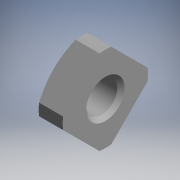
# Autodesk Inventor part: DIN 557 - M4
Saved by Autodesk Inventor 2017.3 (Build 213256000, 256)
## iProperties
Part Number: DIN 557 - M4
Material: Generic
Catalog Web Link: www.cadenas.de
Description: DIN-557-Square nuts
Vendor: FESTO
Document SubType Name: Modeling
Designer: partserver
Manufacturer: FESTO
Mass: 0.122402 g
Surface Area: 1.83702 cm^2
Volume: 0.122402 cm^3
Density: 1 g/cm^3
Appearance: PSOLRGB-192-192-192
Category: PARTsolutions
Company: FESTO
Title: DIN 557 - M4
Author: Cadenas PARTsolutions
Comments: Square nuts
PSOL_IDENT_0: {$CADENAS_DATA\23d-libs\festo\zyl_zubeh\din_557\din_557.prj},178 {VTYP=3D},{NB=DIN 557 - M4},{LINA=D
PSOL_IDENT_1: IN 557 - M4},{NN=DIN-557},{DATE=28.05.2015 11:13:37},{GEOMDATE=10.08.2011 05:48:00},{VERSION=v070619
PSOL_IDENT_2: 081727},{LINEID=10},{WBVAR=},{WBNUMERIC=}  {NB=DIN 557 - M4},{LINA=DIN 557 - M4},{KT=X},{IDNR=},{NEN
PSOL_IDENT_3: N=M4},{D=4.000},{D1=4.134},{P=0.700},{M=3.200},{S=7.000},{SW=},{DW=5.700},{NN=M4}
NB: DIN 557 - M4
NN: M4
NT: Square nuts
NBSYN: DIN 557 - $NENN.
LINA: DIN 557 - M4
CATALOG: Festo
ROWDESC: M4
D: 4
D1: 4.134
P: 0.7
M: 3.2
S: 7
DW: 5.7
SUPPLIER: FESTO
ARTICLENO: DIN 557 - M4
BOMINFO: DIN 557 - M4
CREATOR: CADENAS GmbH
Autodesk Inventor part; units mm, degrees
sketch "Sketch_2" plane through (0, 0, 0) normal (0, 0, 1) x (1, 0, 0)
  line L0 (3.2, 0) -> (0, 0)
  line L1 (0, 0) -> (0, 4.9497)
  line L2 (0, 4.9497) -> (2.287, 4.9497)
  line L3 (2.287, 4.9497) -> (3.2, 2.85)
  line L4 (3.2, 2.85) -> (3.2, 0)
  line L5 (3.2, 0) -> (0, 0)
  constraints: 12 end point
revolve "Revolution1" add sketch "Sketch_2" angle 360 about axis through (3.2, 0, 0) along (1, 0, 0)
sketch "Skizze_2" plane through (0, 0, 0) normal (1, 0, 0) x (0, 1, 0)
  line L0 (14, 14) -> (-14, 14)
  line L1 (-14, 14) -> (-14, -14)
  line L2 (-14, -14) -> (14, -14)
  line L3 (14, -14) -> (14, 14)
  line L4 (0, 5.0205) -> (-5.0205, 0)
  line L5 (-5.0205, 0) -> (0, -5.0205)
  line L6 (0, -5.0205) -> (5.0205, 0)
  line L7 (5.0205, 0) -> (0, 5.0205)
  constraints: 16 end point
extrude "Extrusion1" cut sketch "Skizze_2" along normal blind 3.2
sketch "Sketch_1" plane through (0, 0, 0) normal (0, 0, 1) x (1, 0, 0)
  line L0 (3.2, 0) -> (0, 0)
  line L1 (0, 0) -> (0, 2)
  line L2 (0, 2) -> (0.379, 1.621)
  line L3 (0.379, 1.621) -> (2.821, 1.621)
  line L4 (2.821, 1.621) -> (3.2, 2)
  line L5 (3.2, 2) -> (3.2, 0)
  line L6 (3.2, 0) -> (0, 0)
  constraints: 14 end point
revolve "Revolution2" cut sketch "Sketch_1" angle 360 about axis through (3.2, 0, 0) along (1, 0, 0)
sketch "Sketch_3" plane through (0, 0, 0) normal (1, 0, 0) x (0, 1, 0)
  line L0 (7, 7) -> (-7, 7)
  line L1 (-7, 7) -> (-7, -7)
  line L2 (-7, -7) -> (7, -7)
  line L3 (7, -7) -> (7, 7)
  circle A0 centre (0, 0) radius 4.45
  constraints: 8 end point, 1 centre point
extrude "Extrusion2" cut sketch "Sketch_3" along normal blind 3.2
ref_plane "IP1_XY" through (0, 0, 0) normal (1, 0, 0) x (0, 0, -1)
ref_plane "IP1_YZ" through (0, 0, 0) normal (0, 0, -1) x (0, 1, 0)
ref_plane "IP1_ZX" through (0, 0, 0) normal (0, 1, 0) x (1, 0, 0)
ref_plane "IP2_XY" through (3.2, 0, 0) normal (1, 0, 0) x (0, 0, -1)
ref_plane "IP2_YZ" through (3.2, 0, 0) normal (0, 0, -1) x (0, 1, 0)
ref_plane "IP2_ZX" through (3.2, 0, 0) normal (0, 1, 0) x (1, 0, 0)
body "Solid1"
